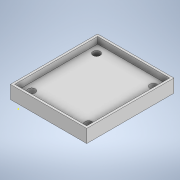
# Autodesk Inventor part: testing holes for circuit board
Saved by Autodesk Inventor 2020.2 (Build 242310000, 310)
## iProperties
Created: 2020-02-12
Part Number: testing holes for circuit board
Material: Generic
Document SubType Name: Modeling
Designer: ColinP
Density: 1 g/cm^3
Appearance: Default
Author: ColinP
Autodesk Inventor part; units mm, degrees
ref_plane "YZ Plane" through (0, 0, 0) normal (1, 0, 0) x (0, 1, 0)
ref_plane "XZ Plane" through (0, 0, 0) normal (0, 1, 0) x (-1, 0, 0)
ref_plane "XY Plane" through (0, 0, 0) normal (0, 0, 1) x (1, 0, 0)
sketch "Sketch1" plane through (0, 0, 0) normal (0, 1, 0) x (-1, 0, 0)
  line L0 (4.6706, 7.7326) -> (-28.3294, 7.7326)
  line L1 (-28.3294, 7.7326) -> (-28.3294, -32.2674)
  line L2 (-28.3294, -32.2674) -> (4.6706, -32.2674)
  line L3 (4.6706, -32.2674) -> (4.6706, 7.7326)
  point P0 (0, 0)
  dimension "d0" = 33
  dimension "d1" = 40
  constraints: 8 end point, 2 parallel, 1 horizontal, 1 perpendicular
  measures "d0" distance of L2.end L1.end
  measures "d1" distance of L1.end L0.end
extrude "Extrusion1" add sketch "Sketch1" along normal blind 3
sketch "Sketch2" plane through (0, 3, 0) normal (0, 1, 0) x (1, 0, 0)
  line L0 (-4.6706, 32.2674) -> (-4.6706, -7.7326) projected
  line L1 (-4.6706, -7.7326) -> (-4.6706, -4.7326)
  line L2 (-4.6706, -4.7326) -> (-2.8206, -4.7326)
  line L3 (-2.8206, -4.7326) -> (-2.8206, 28.2674)
  line L4 (-2.8206, 28.2674) -> (26.4794, 28.2674)
  line L5 (26.4794, 28.2674) -> (26.4794, -4.7326)
  line L6 (-2.8206, -4.7326) -> (-1.1706, -4.7326)
  line L7 (26.4794, -4.7326) -> (24.8794, -4.7326)
  line L8 (24.8794, -4.7326) -> (24.8794, 28.2674)
  line L9 (-2.8206, 28.2674) -> (-1.1706, 28.2674)
  line L10 (-1.1706, -4.7326) -> (-1.1706, -1.4326)
  line L11 (-1.1706, -1.4326) -> (24.8794, -1.4326)
  point P0 (0, 0)
  dimension "d4" = 3
  dimension "d5" = 1.85
  dimension "d6" = 90
  dimension "d7" = 33
  dimension "d8" = 29.3
  dimension "d9" = 1.65
  dimension "d10" = 1.6
  dimension "d11" = 1.65
  dimension "d26" = 3.3
  constraints: 22 end point, 6 perpendicular, 5 point on line, 2 horizontal, 1 vertical
  measures "d4" distance of L0.end L1.end
  measures "d5" distance of L1.end L2.end
  measures "d6" angle of L1 L2
  measures "d7" distance of L2.end L3.end
  measures "d8" distance of L3.end L4.end
  measures "d9" distance of L2.end L6.end
  measures "d10" distance of L5.end L7.end
  measures "d11" distance of L3.end L9.end
  measures "d26" distance of L6.end L10.end
hole "Hole1" at (-1.1706, 3, 1.4326) at (24.8794, 3, 1.4326) at (24.8794, 3, -28.2674) at (-1.1706, 3, -28.2674) direction (0, -1, 0) diameter 3.3 end through all
sketch "Sketch3" plane through (0, 0, 0) normal (0, -1, 0) x (1, 0, 0)
  line L0 (28.3294, -32.2674) -> (-4.6706, -32.2674) projected
  line L1 (-4.6706, -32.2674) -> (-5.6706, -32.2674)
  line L2 (-5.6706, -32.2674) -> (-5.6706, -33.2674)
  line L3 (-5.6706, -33.2674) -> (29.3294, -33.2674)
  line L4 (29.3294, -33.2674) -> (29.3294, 8.7326)
  line L5 (28.3294, 7.7326) -> (28.3294, -32.2674) projected
  line L6 (29.3294, 8.7326) -> (-5.6706, 8.7326)
  line L7 (-5.6706, 8.7326) -> (-5.6706, -32.2674)
  circle A0 centre (24.8794, -28.2674) radius 1.65 projected
  circle A1 centre (-1.1706, -28.2674) radius 1.65 projected
  line L8 (-4.6706, 7.7326) -> (28.3294, 7.7326) projected
  line L9 (-4.6706, -32.2674) -> (-4.6706, 7.7326) projected
  line L10 (28.3294, -32.2674) -> (-4.6706, -32.2674) projected
  line L11 (28.3294, 7.7326) -> (28.3294, -32.2674) projected
  point P0 (0, 0)
  dimension "d19" = 1
  dimension "d20" = 1
  dimension "d21" = 35
  dimension "d22" = 42
  dimension "d23" = 90
  constraints: 12 end point, 4 perpendicular, 1 horizontal, 1 parallel, 1 point on line
  measures "d19" distance of L0.end L1.end
  measures "d20" distance of L1.end L2.end
  measures "d21" distance of L2.end L3.end
  measures "d22" distance of L3.end L4.end
  measures "d23" angle of L4 L3
extrude "Extrusion2" add sketch "Sketch3" against normal blind 6 contours L7 L6 L4 L3 L2
sketch "Sketch4" plane through (-5.6706, 0, 8.7326) normal (0, 0, 1) x (1, 0, 0)
  point P0 (5.6706, 0)
sketch "Sketch5" plane through (0, 0, 0) normal (0, -1, 0) x (1, 0, 0)
  line L0 (-5.6706, -33.2674) -> (-5.6706, 8.7326) projected
  line L1 (-5.6706, 8.7326) -> (-5.6706, 5.7326)
  line L2 (-5.6706, 5.7326) -> (29.3294, 5.7326)
  line L3 (29.3294, -33.2674) -> (29.3294, 8.7326) projected
  line L4 (29.3294, 8.7326) -> (-5.6706, 8.7326)
  line L5 (-5.6706, 5.7326) -> (-5.6706, 6.7326)
  line L6 (-5.6706, 6.7326) -> (29.3294, 6.7326)
  line L7 (28.3294, 7.7326) -> (-4.6706, 7.7326) projected
  line L8 (29.3294, 6.7326) -> (29.3294, 5.7326)
  point P0 (0, 0)
  dimension "d27" = 3
  dimension "d28" = 1
  constraints: 12 end point, 3 point on line, 2 parallel, 2 perpendicular
  measures "d27" distance of L0.end L1.end
  measures "d28" distance of L1.end L5.end
extrude "Extrusion3" cut sketch "Sketch5" against normal blind 10 contours L0 L4 L3 L6
extrude "Extrusion4" add sketch "Sketch5" against normal blind 6 contours L0 L6 L3 L2
body "Solid1"
